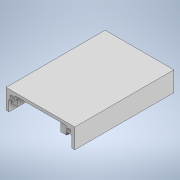
# Autodesk Inventor part: Caja1
Saved by Autodesk Inventor 2021 (Build 250183000, 183)
## iProperties
Created: 2021-02-21
Part Number: Caja1
Material: Generic
Document SubType Name: Modeling
Designer: deuts
Density: 1 g/cm^3
Appearance: Default
Author: deuts
Autodesk Inventor part; units mm, degrees
ref_plane "YZ Plane" through (0, 0, 0) normal (1, 0, 0) x (0, 1, 0)
ref_plane "XZ Plane" through (0, 0, 0) normal (0, 1, 0) x (-1, 0, 0)
ref_plane "XY Plane" through (0, 0, 0) normal (0, 0, 1) x (1, 0, 0)
sketch "Sketch1" plane through (0, 0, 0) normal (0, 1, 0) x (-1, 0, 0)
  line L0 (55, -86.5) -> (-55, -86.5)
  line L1 (-55, -86.5) -> (-55, 86.5)
  line L2 (-55, 86.5) -> (55, 86.5)
  line L3 (55, 86.5) -> (55, -86.5)
  line L4 (55, -86.5) -> (-55, 86.5) construction
  line L5 (-55, -86.5) -> (55, 86.5) construction
  point P0 (0, 0)
  dimension "d0" = 110
  dimension "d1" = 173
  constraints: 12 end point, 2 midpoint, 2 parallel, 1 horizontal, 1 perpendicular
  measures "d0" distance of L1.end L2.end
  measures "d1" distance of L0.end L1.end
extrude "Extrusion1" add sketch "Sketch1" along normal blind 5
sketch "Sketch2" plane through (0, 5, 0) normal (0, 1, 0) x (1, 0, 0)
  line L0 (-55, -86.5) -> (55, -86.5) projected
  line L1 (-55, -86.5) -> (-60, -86.5)
  line L2 (-60, -86.5) -> (-60, 86.5)
  line L3 (-60, 86.5) -> (-55, 86.5)
  line L4 (-55, 86.5) -> (-55, -86.5)
  point P0 (0, 0)
  dimension "d4" = 5
  constraints: 8 end point, 2 parallel, 1 horizontal, 1 perpendicular
  measures "d4" distance of L2.end L3.end
extrude "Extrusion2" add sketch "Sketch2" against normal blind 34.5
sketch "Sketch3" plane through (0, 5, 0) normal (0, 1, 0) x (1, 0, 0)
  line L0 (55, -86.5) -> (55, 86.5) projected
  line L1 (55, -86.5) -> (60, -86.5)
  line L2 (60, -86.5) -> (60, 86.5)
  line L3 (60, 86.5) -> (55, 86.5)
  line L4 (55, 86.5) -> (55, -86.5)
  point P0 (0, 0)
  dimension "d7" = 5
  constraints: 8 end point, 2 parallel, 1 horizontal, 1 perpendicular
  measures "d7" distance of L3.end L2.end
extrude "Extrusion3" add sketch "Sketch3" against normal blind 34.5
sketch "Sketch4" plane through (-60, -29.5, 86.5) normal (0, 0, 1) x (1, 0, 0)
  line L0 (5, 29.5) -> (5, 0) projected
  line L1 (5, 29.5) -> (15, 29.5)
  line L2 (15, 29.5) -> (15, 19.5)
  line L3 (15, 19.5) -> (5, 19.5)
  line L4 (5, 19.5) -> (5, 29.5)
  circle A0 centre (10, 24.5) radius 3
  point P0 (60, 29.5)
  point P1 (5, 19.5)
  dimension "d10" = 10
  dimension "d11" = 10
  dimension "d23" = 5
  dimension "d24" = 5
  dimension "d26" = 6
  constraints: 8 end point, 2 parallel, 1 centre point, 1 horizontal, 1 perpendicular
  measures "d10" distance of L2.end L3.end
  measures "d11" distance of L1.end L2.end
  measures "d23" horizontal distance of L2.end A0.centre
  measures "d24" horizontal distance of L1.end A0.centre
  measures "d26" diameter of A0
extrude "Extrusion4" add sketch "Sketch4" against normal blind 5
pattern_linear "Rectangular Pattern1" count 2 spacing 100 along (1, 0, 0) count 2 spacing 168 along (0, 0, -1) of "Extrusion4"
fillet "Fillet3" radius 2 12 edges at (-55, -10, 84) (-45, -10, 84) (-45, 0, 84) (45, -10, 84) (55, -10, 84) (45, 0, 84) (45, -10, -84) (55, -10, -84) (45, 0, -84) (-55, -10, -84) (-45, -10, -84) (-45, 0, -84)
sketch "Sketch7" plane through (-60, 5, -86.5) normal (-1, 0, 0) x (0, 0, 1)
  line L0 (53, -16.5) -> (40, -16.5)
  line L1 (40, -16.5) -> (40, -25.5)
  line L2 (40, -25.5) -> (53, -25.5)
  line L3 (53, -25.5) -> (53, -16.5)
  line L4 (53, -16.5) -> (40, -25.5) construction
  line L5 (40, -16.5) -> (53, -25.5) construction
  line L6 (0, 0) -> (0, -34.5) projected
  line L7 (173, -34.5) -> (0, -34.5) projected
  point P0 (86.5, -5)
  point P1 (46.5, -21)
  dimension "d33" = 9
  dimension "d34" = 13
  dimension "d35" = 40
  constraints: 12 end point, 2 midpoint, 2 parallel, 1 horizontal, 1 perpendicular
  measures "d33" distance of L2.end L0.start
  measures "d34" distance of L0.start L0.end
  measures "d35" distance from line of L6 L1.end
extrude "Extrusion6" cut sketch "Sketch7" against normal blind 5
sketch "Sketch8" plane through (0, 0, 0) normal (0, -1, 0) x (1, 0, 0)
  circle A0 centre (-50, 76.5) radius 1.25
  line L0 (-47, 81.5) -> (-53, 81.5) projected
  line L1 (-55, -86.5) -> (-55, 86.5) projected
  line L2 (-55, 71.5) -> (-45, 71.5)
  line L3 (-45, 71.5) -> (-45, 81.5)
  line L4 (-45, 81.5) -> (-55, 81.5)
  line L5 (-55, 81.5) -> (-55, 71.5)
  line L6 (-55, 71.5) -> (-45, 81.5) construction
  line L7 (-45, 71.5) -> (-55, 81.5) construction
  point P0 (0, 0)
  dimension "d39" = 2.5
  dimension "d40" = 5
  dimension "d41" = 5
  dimension "d42" = 10
  dimension "d43" = 10
  constraints: 12 end point, 2 midpoint, 2 parallel, 1 centre point, 1 horizontal, 1 perpendicular
  measures "d39" diameter of A0
  measures "d40" distance from line of L0 A0.centre
  measures "d41" distance from line of L1 A0.centre
  measures "d42" distance of L2.end L3.end
  measures "d43" distance of L2.start L2.end
extrude "Extrusion7" add sketch "Sketch8" along normal blind 19.5 contours A0 | L4 L3 L2 L1 L0
pattern_linear "Rectangular Pattern2" count 2 spacing 85.8 along (1, 0, 0) count 2 spacing 57.4 along (0, 0, -1) of "Extrusion7"
body "Solid1"
